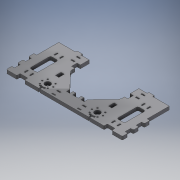
# Autodesk Inventor part: Bulkhead
Saved by Autodesk Inventor 2016 (Build 200138000, 138)
## iProperties
Created: 2014-06-30
Part Number: Bulkhead
Material: Generic
Document SubType Name: Modeling
Designer: STACKPOLE
Density: 1 g/cm^3
Appearance: Default
Author: STACKPOLE
Autodesk Inventor part; units mm, degrees
ref_plane "YZ Plane" through (0, 0, 0) normal (1, 0, 0) x (0, 1, 0)
ref_plane "XZ Plane" through (0, 0, 0) normal (0, 1, 0) x (-1, 0, 0)
ref_plane "XY Plane" through (0, 0, 0) normal (0, 0, 1) x (1, 0, 0)
sketch "Sketch1" plane through (0, 0, 0) normal (0, 0, 1) x (1, 0, 0)
  line L0 (0, -90) -> (-103, -90)
  line L1 (0, 0) -> (0, -90) construction
  line L2 (-105, -88) -> (-105, -82)
  line L3 (-103, -80) -> (-100, -80)
  line L4 (-100, -70) -> (-103, -70)
  line L5 (-105, -68) -> (-105, -62)
  line L6 (-103, -60) -> (-100, -60)
  line L7 (-100, -80) -> (-100, -70)
  line L8 (-100, -50) -> (-103, -50)
  line L9 (-105, -48) -> (-105, -42)
  line L10 (-103, -40) -> (-100, -40)
  line L11 (-100, -60) -> (-100, -50)
  line L12 (-100, -40) -> (-100, 0)
  line L13 (-70, 0) -> (-70, 3)
  line L14 (-70, 3) -> (-60, 3)
  line L15 (-60, 3) -> (-60, 0)
  line L16 (-100, 0) -> (-70, 0)
  line L17 (-60, 0) -> (-45, 0)
  line L18 (-45, 0) -> (-45, -29.9568)
  arc A0 (-105, -88) -> (-103, -90) centre (-103, -88) ccw
  arc A1 (-103, -80) -> (-105, -82) centre (-103, -82) ccw
  arc A2 (-105, -68) -> (-103, -70) centre (-103, -68) ccw
  arc A3 (-103, -60) -> (-105, -62) centre (-103, -62) ccw
  arc A4 (-105, -48) -> (-103, -50) centre (-103, -48) ccw
  arc A5 (-103, -40) -> (-105, -42) centre (-103, -42) ccw
  line L19 (0, -90) -> (103, -90)
  line L20 (105, -88) -> (105, -82)
  line L21 (103, -80) -> (100, -80)
  line L22 (100, -70) -> (103, -70)
  line L23 (105, -68) -> (105, -62)
  line L24 (103, -60) -> (100, -60)
  line L25 (100, -80) -> (100, -70)
  line L26 (100, -50) -> (103, -50)
  line L27 (105, -48) -> (105, -42)
  line L28 (103, -40) -> (100, -40)
  line L29 (100, -60) -> (100, -50)
  line L30 (100, -40) -> (100, 0)
  line L31 (70, 0) -> (70, 3)
  line L32 (70, 3) -> (60, 3)
  line L33 (60, 3) -> (60, 0)
  line L34 (100, 0) -> (70, 0)
  line L35 (60, 0) -> (45, 0)
  line L36 (45, 0) -> (45, -29.9568)
  arc A6 (103, -90) -> (105, -88) centre (103, -88) ccw
  arc A7 (105, -82) -> (103, -80) centre (103, -82) ccw
  arc A8 (103, -70) -> (105, -68) centre (103, -68) ccw
  arc A9 (105, -62) -> (103, -60) centre (103, -62) ccw
  arc A10 (103, -50) -> (105, -48) centre (103, -48) ccw
  arc A11 (105, -42) -> (103, -40) centre (103, -42) ccw
  line L37 (-42.1899, -36.907) -> (-16, -64)
  line L38 (16, -64) -> (42.1899, -36.907)
  line L39 (-16, -70) -> (-10, -70)
  line L40 (-10, -70) -> (-10, -64)
  line L41 (-5, -64) -> (-5, -70)
  line L42 (-5, -70) -> (5, -70)
  line L43 (5, -70) -> (5, -64)
  line L44 (10, -64) -> (10, -70)
  line L45 (10, -70) -> (16, -70)
  line L46 (-10, -64) -> (-5, -64)
  line L47 (5, -64) -> (10, -64)
  line L48 (16, -64) -> (16, -70)
  line L49 (-16, -64) -> (-16, -70)
  arc A12 (-45, -29.9568) -> (-42.1899, -36.907) centre (-35, -29.9568) ccw
  arc A13 (42.1899, -36.907) -> (45, -29.9568) centre (35, -29.9568) ccw
  point P0 (-105, -90)
  point P1 (-105, -80)
  point P2 (-105, -70)
  point P3 (-105, -60)
  point P4 (-105, -50)
  point P5 (-105, -40)
  point P6 (105, -90)
  point P7 (105, -80)
  point P8 (105, -70)
  point P9 (105, -60)
  point P10 (105, -50)
  point P11 (105, -40)
  point P12 (-45, -34)
  point P13 (45, -34)
  point P14 (0, -70)
  dimension "d4" = 105
  dimension "d5" = 10
  dimension "d6" = 5
  dimension "d8" = 10
  dimension "d9" = 10
  dimension "d10" = 10
  dimension "d11" = 10
  dimension "d12" = 30
  dimension "d13" = 10
  dimension "d14" = 3
  dimension "d15" = 90
  dimension "d18" = 15
  dimension "d19" = 34
  dimension "d20" = 2
  dimension "d102" = 5
  dimension "d104" = 5
  dimension "d105" = 10
  dimension "d160" = 6
  dimension "d161" = 6
  dimension "d162" = 6
  dimension "d163" = 70
  dimension "d175" = 10
  constraints: 100 end point, 36 symmetric about line, 28 point on circle, 28 point on line, 23 perpendicular, 16 tangent, 14 centre point, 10 parallel, 6 equal radius, 6 horizontal alignment, 5 vertical alignment, 2 horizontal, 1 midpoint, 1 vertical, 6 other
  measures "d4" distance of L0.start point (-105, -90)
  measures "d5" distance of point (-105, -90) point (-105, -80)
  measures "d6" distance of point (-105, -80) L3.end
  measures "d8" distance between parallel lines of L3 L4
  measures "d9" distance of point (-105, -70) point (-105, -60)
  measures "d10" distance between parallel lines of L6 L8
  measures "d11" distance of point (-105, -50) point (-105, -40)
  measures "d12" distance from line of L12 L13.start
  measures "d13" distance of L13.end L14.end
  measures "d14" distance of L13.start L13.end
  measures "d15" distance between parallel lines of L16 L0
  measures "d18" distance of L15.end L17.end
  measures "d19" distance of point (-45, -34) L17.end
  measures "d20" radius of A0
  measures "d102" distance between parallel lines of L41 L40
  measures "d104" distance between parallel lines of L44 L43
  measures "d105" distance between parallel lines of L41 L43
  measures "d160" distance of L37.end L39.start
  measures "d161" distance of L39.start L39.end
  measures "d162" distance of L44.end L45.end
  measures "d163" distance between parallel lines of L35 L42
  measures "d175" radius of A12
extrude "Extrusion1" add sketch "Sketch1" along normal blind 6
sketch "Sketch2" plane through (0, 0, 6) normal (0, 0, 1) x (1, 0, 0)
  line L0 (-103, -90) -> (103, -90) projected
  line L1 (-70, 0) -> (-100, 0) projected
  circle A0 centre (-45, -75) radius 5
  circle A1 centre (-45, -75) radius 10 construction
  line L2 (-45, -75) -> (-52.0711, -67.9289) construction
  line L3 (-45, -75) -> (-55, -75) construction
  line L4 (-55, -75) -> (-45, -75) construction
  circle A2 centre (-52.0711, -67.9289) radius 1.25
  circle A3 centre (-55, -75) radius 1.25
  circle A4 centre (-52.0711, -82.0711) radius 1.25
  line L5 (-45, -65) -> (-45, -85) construction
  circle A5 centre (-37.9289, -67.9289) radius 1.25
  circle A6 centre (-35, -75) radius 1.25
  circle A7 centre (-37.9289, -82.0711) radius 1.25
  line L6 (0, 0) -> (0, -90) construction
  circle A8 centre (45, -75) radius 5
  circle A9 centre (45, -75) radius 10 construction
  line L7 (45, -75) -> (52.0711, -67.9289) construction
  line L8 (45, -75) -> (55, -75) construction
  line L9 (55, -75) -> (45, -75) construction
  circle A10 centre (52.0711, -67.9289) radius 1.25
  circle A11 centre (55, -75) radius 1.25
  circle A12 centre (52.0711, -82.0711) radius 1.25
  line L10 (45, -65) -> (45, -85) construction
  circle A13 centre (37.9289, -67.9289) radius 1.25
  circle A14 centre (35, -75) radius 1.25
  circle A15 centre (37.9289, -82.0711) radius 1.25
  dimension "d23" = 10
  dimension "d25" = 75
  dimension "d26" = 45
  dimension "d27" = 20
  dimension "d28" = 45
  dimension "d29" = 2.5
  dimension "d30" = 2.5
  constraints: 18 end point, 16 centre point, 16 symmetric about line, 8 point on circle, 6 coincident, 1 collinear, 1 midpoint, 1 parallel, 1 perpendicular, 12 other
  measures "d23" diameter of A0
  measures "d25" vertical distance of A0.centre L6.start
  measures "d26" horizontal distance of L6.start A0.centre
  measures "d27" diameter of A1
  measures "d28" angle of L4 L2
  measures "d29" diameter of A2
  measures "d30" diameter of A3
extrude "Extrusion2" cut sketch "Sketch2" against normal blind 6
sketch "Sketch3" plane through (0, 0, 6) normal (0, 0, 1) x (1, 0, 0)
  line L0 (-103, -90) -> (103, -90) projected
  line L1 (-70, 0) -> (-100, 0) projected
  line L2 (-85, -18) -> (-83, -18)
  line L3 (-83, -18) -> (-83, -24)
  line L4 (-83, -24) -> (-85, -24)
  line L5 (-85, -24) -> (-85, -18)
  line L6 (-75, -18) -> (-73, -18)
  line L7 (-73, -18) -> (-73, -24)
  line L8 (-73, -24) -> (-75, -24)
  line L9 (-75, -24) -> (-75, -18)
  line L10 (0, 0) -> (0, -90) construction
  line L11 (85, -18) -> (83, -18)
  line L12 (83, -18) -> (83, -24)
  line L13 (83, -24) -> (85, -24)
  line L14 (85, -24) -> (85, -18)
  line L15 (75, -18) -> (73, -18)
  line L16 (73, -18) -> (73, -24)
  line L17 (73, -24) -> (75, -24)
  line L18 (75, -24) -> (75, -18)
  line L19 (-100, 0) -> (-100, -40) projected
  line L20 (-75, -21) -> (-83, -21) construction
  line L21 (-73, -78) -> (-75, -78)
  line L22 (-75, -78) -> (-75, -72)
  line L23 (-75, -72) -> (-73, -72)
  line L24 (-73, -72) -> (-73, -78)
  line L25 (-85, -72) -> (-83, -72)
  line L26 (-83, -72) -> (-83, -78)
  line L27 (-83, -78) -> (-85, -78)
  line L28 (-85, -78) -> (-85, -72)
  line L29 (73, -78) -> (75, -78)
  line L30 (75, -78) -> (75, -72)
  line L31 (75, -72) -> (73, -72)
  line L32 (73, -72) -> (73, -78)
  line L33 (85, -72) -> (83, -72)
  line L34 (83, -72) -> (83, -78)
  line L35 (83, -78) -> (85, -78)
  line L36 (85, -78) -> (85, -72)
  line L37 (-45, -29.9568) -> (-45, 0) projected
  line L38 (-55.5, -17) -> (-61.5, -17)
  line L39 (-61.5, -17) -> (-61.5, -15)
  line L40 (-61.5, -15) -> (-55.5, -15)
  line L41 (-55.5, -15) -> (-55.5, -17)
  line L42 (-55.5, -7) -> (-61.5, -7)
  line L43 (-61.5, -7) -> (-61.5, -5)
  line L44 (-61.5, -5) -> (-55.5, -5)
  line L45 (-55.5, -5) -> (-55.5, -7)
  line L46 (55.5, -17) -> (61.5, -17)
  line L47 (61.5, -17) -> (61.5, -15)
  line L48 (61.5, -15) -> (55.5, -15)
  line L49 (55.5, -15) -> (55.5, -17)
  line L50 (55.5, -7) -> (61.5, -7)
  line L51 (61.5, -7) -> (61.5, -5)
  line L52 (61.5, -5) -> (55.5, -5)
  line L53 (55.5, -5) -> (55.5, -7)
  point P0 (-79, -21)
  dimension "d41" = 6
  dimension "d43" = 18
  dimension "d129" = 15
  dimension "d130" = 8
  dimension "d131" = 2
  dimension "d132" = 2
  dimension "d219" = 12
  dimension "d314" = 5
  dimension "d316" = 8
  dimension "d317" = 10.5
  constraints: 100 end point, 24 symmetric about line, 12 parallel, 7 equal length, 6 horizontal, 6 perpendicular, 4 midpoint, 4 point on line, 3 collinear, 2 horizontal alignment
  measures "d41" distance of L4.end L2.start
  measures "d43" distance between parallel lines of L1 L2
  measures "d129" distance between parallel lines of L5 L19
  measures "d130" distance between parallel lines of L9 L3
  measures "d131" distance of L6.start L6.end
  measures "d132" distance of L2.start L2.end
  measures "d219" distance between parallel lines of L0 L27
  measures "d314" distance between parallel lines of L1 L44
  measures "d316" distance between parallel lines of L42 L40
  measures "d317" distance between parallel lines of L37 L41
sketch "Sketch8" plane through (0, 0, 6) normal (0, 0, 1) x (1, 0, 0)
  line L0 (-45, -29.9568) -> (-45, 0) projected
  line L1 (-45, -16) -> (-51, -16)
  line L2 (-51, -16) -> (-51, -26)
  line L3 (-51, -26) -> (-45, -26)
  line L4 (-45, -26) -> (-45, -16)
  line L5 (-45, 0) -> (-60, 0) projected
  line L6 (-45, -45) -> (-51, -45)
  line L7 (-51, -45) -> (-51, -55)
  line L8 (-51, -55) -> (-45, -55)
  line L9 (-45, -55) -> (-45, -45)
  line L10 (45, 0) -> (45, -29.9568) projected
  line L11 (45, -16) -> (51, -16)
  line L12 (51, -16) -> (51, -26)
  line L13 (51, -26) -> (45, -26)
  line L14 (45, -26) -> (45, -16)
  line L15 (45, -45) -> (51, -45)
  line L16 (51, -45) -> (51, -55)
  line L17 (51, -55) -> (45, -55)
  line L18 (45, -55) -> (45, -45)
  point P0 (0, 0)
  dimension "d177" = 6
  dimension "d178" = 10
  dimension "d179" = 16
  dimension "d180" = 10
  dimension "d181" = 6
  dimension "d182" = 55
  dimension "d183" = 6
  dimension "d184" = 10
  constraints: 32 end point, 8 parallel, 4 horizontal, 4 perpendicular, 3 horizontal alignment, 3 vertical alignment, 2 point on line
  measures "d177" distance of L1.start L1.end
  measures "d178" distance of L1.end L2.end
  measures "d179" distance between parallel lines of L5 L1
  measures "d180" distance of L6.end L7.end
  measures "d181" distance of L7.end L8.end
  measures "d182" distance between parallel lines of L5 L8
  measures "d183" distance of L11.start L11.end
  measures "d184" distance of L11.end L12.end
extrude "Extrusion16" cut sketch "Sketch8" against normal through all
sketch "Sketch9" plane through (0, 0, 6) normal (0, 0, 1) x (1, 0, 0)
  circle A0 centre (45, -75) radius 5 construction
  circle A1 centre (45, -75) radius 8.75 construction
  circle A2 centre (45, -75) radius 11.5 construction
  circle A3 centre (37.9289, -82.0711) radius 1.25 construction
  line L0 (-103, -90) -> (103, -90) construction
  line L1 (0, -90) -> (0, 0) construction
  line L2 (51, -45) -> (51, -55) projected
  arc A4 (40.8921, -82.7258) -> (49.1079, -82.7258) centre (45, -75) ccw
  line L3 (49.1079, -82.7258) -> (50.3989, -85.1539)
  line L4 (40.8921, -82.7258) -> (39.6011, -85.1539)
  line L5 (-103, -90) -> (103, -90) projected
  line L6 (45, -75) -> (45, -59.2152) construction
  line L7 (46.15, -90) -> (46.15, -86.4424)
  line L8 (43.85, -90) -> (43.85, -86.4424)
  arc A5 (39.6011, -85.1539) -> (43.85, -86.4424) centre (45, -75) ccw
  arc A6 (46.15, -86.4424) -> (50.3989, -85.1539) centre (45, -75) ccw
  line L9 (46.15, -90) -> (43.85, -90)
  circle A7 centre (-45, -75) radius 5 construction
  circle A8 centre (-45, -75) radius 8.75 construction
  circle A9 centre (-45, -75) radius 11.5 construction
  circle A10 centre (-37.9289, -82.0711) radius 1.25 construction
  line L10 (-51, -45) -> (-51, -55)
  arc A11 (-49.1079, -82.7258) -> (-40.8921, -82.7258) centre (-45, -75) ccw
  line L11 (-49.1079, -82.7258) -> (-50.3989, -85.1539)
  line L12 (-40.8921, -82.7258) -> (-39.6011, -85.1539)
  line L13 (-45, -75) -> (-45, -59.2152) construction
  line L14 (-46.15, -90) -> (-46.15, -86.4424)
  line L15 (-43.85, -90) -> (-43.85, -86.4424)
  arc A12 (-43.85, -86.4424) -> (-39.6011, -85.1539) centre (-45, -75) ccw
  arc A13 (-50.3989, -85.1539) -> (-46.15, -86.4424) centre (-45, -75) ccw
  line L16 (-46.15, -90) -> (-43.85, -90)
  point P0 (77, -74)
  point P1 (79, -74)
  point P2 (46.7957, -86.3589)
  point P3 (44, -86.4564)
  point P4 (-46.7957, -86.3589)
  point P5 (-44, -86.4564)
  dimension "d191" = 23
  dimension "d239" = 56
  dimension "d288" = 28
  dimension "d289" = 2.3
  dimension "d290" = 1.15
  constraints: 28 end point, 28 point on circle, 19 symmetric about line, 12 centre point, 4 coincident, 4 line through centre, 2 point on line, 2 vertical, 1 collinear, 1 concentric, 1 midpoint, 1 parallel, 1 perpendicular, 1 tangent, 7 other
  measures "d191" diameter of A2
  measures "d239" angle of L4 L3
  measures "d288" angle of L6 L4
  measures "d289" distance between parallel lines of L8 L7
  measures "d290" distance between parallel lines of L8 L6
extrude "Extrusion31" cut sketch "Sketch3" against normal through all
extrude "Extrusion32" cut sketch "Sketch9" against normal blind 10
sketch "Sketch20" plane through (0, 0, 6) normal (0, 0, 1) x (1, 0, 0)
  line L0 (0, 0) -> (0, -123) construction
  line L1 (-20, -87) -> (-26, -87)
  line L2 (-26, -87) -> (-26, -85)
  line L3 (-26, -85) -> (-20, -85)
  line L4 (-20, -85) -> (-20, -87)
  line L5 (-20, -78) -> (-26, -78)
  line L6 (-26, -78) -> (-26, -76)
  line L7 (-26, -76) -> (-20, -76)
  line L8 (-20, -76) -> (-20, -78)
  line L9 (-43.85, -90) -> (43.85, -90) projected
  line L10 (20, -87) -> (26, -87)
  line L11 (26, -87) -> (26, -85)
  line L12 (26, -85) -> (20, -85)
  line L13 (20, -85) -> (20, -87)
  line L14 (20, -78) -> (26, -78)
  line L15 (26, -78) -> (26, -76)
  line L16 (26, -76) -> (20, -76)
  line L17 (20, -76) -> (20, -78)
  dimension "d293" = 2
  dimension "d294" = 2
  dimension "d295" = 7
  dimension "d296" = 6
  dimension "d297" = 3
  dimension "d298" = 20
  constraints: 34 end point, 8 symmetric about line, 4 parallel, 2 horizontal, 2 perpendicular, 2 point on line, 1 collinear, 1 vertical
  measures "d293" distance of L1.end L2.end
  measures "d294" distance of L5.end L6.end
  measures "d295" distance between parallel lines of L5 L3
  measures "d296" distance of L1.start L1.end
  measures "d297" distance between parallel lines of L9 L1
  measures "d298" distance between parallel lines of L0 L4
extrude "Extrusion33" cut sketch "Sketch20" against normal blind 10
sketch "Sketch21" plane through (0, 0, 6) normal (0, 0, 1) x (1, 0, 0)
  line L0 (83, -67) -> (75, -67)
  line L1 (72, -64) -> (72, -32)
  line L2 (75, -29) -> (83, -29)
  line L3 (86, -32) -> (86, -64)
  line L4 (85, -72) -> (85, -78) projected
  line L5 (73, -78) -> (73, -72) projected
  line L6 (75, -72) -> (73, -72) projected
  line L7 (75, -24) -> (73, -24) projected
  arc A0 (83, -67) -> (86, -64) centre (83, -64) ccw
  arc A1 (72, -64) -> (75, -67) centre (75, -64) ccw
  arc A2 (75, -29) -> (72, -32) centre (75, -32) ccw
  arc A3 (86, -32) -> (83, -29) centre (83, -32) ccw
  line L8 (0, 0) -> (0, -90) construction
  line L9 (-43.85, -90) -> (43.85, -90) construction
  line L10 (-83, -67) -> (-75, -67)
  line L11 (-72, -64) -> (-72, -32)
  line L12 (-75, -29) -> (-83, -29)
  line L13 (-86, -32) -> (-86, -64)
  arc A4 (-86, -64) -> (-83, -67) centre (-83, -64) ccw
  arc A5 (-75, -67) -> (-72, -64) centre (-75, -64) ccw
  arc A6 (-72, -32) -> (-75, -29) centre (-75, -32) ccw
  arc A7 (-83, -29) -> (-86, -32) centre (-83, -32) ccw
  line L14 (83, -72) -> (83, -78) construction
  line L15 (83, -75) -> (75, -75) construction
  line L16 (75, -72) -> (75, -78) construction
  point P0 (79, -67)
  point P1 (79, -75)
  dimension "d301" = 5
  dimension "d302" = 5
  dimension "d303" = 3
  dimension "d310" = 14
  constraints: 20 end point, 16 point on circle, 12 symmetric about line, 8 centre point, 8 tangent, 5 midpoint, 3 equal radius, 2 parallel, 1 horizontal, 1 perpendicular, 1 vertical alignment, 4 other
  measures "d301" distance between parallel lines of L6 L0
  measures "d302" distance between parallel lines of L7 L2
  measures "d303" radius of A0
  measures "d310" distance between parallel lines of L1 L3
extrude "Extrusion34" cut sketch "Sketch21" against normal through all
sketch "Sketch22" plane through (0, 0, 6) normal (0, 0, 1) x (1, 0, 0)
  line L0 (46.15, -90) -> (103, -90) projected
  line L1 (86, -90) -> (86, -84)
  line L2 (86, -84) -> (72, -84)
  line L3 (72, -84) -> (72, -90)
  line L4 (-103, -90) -> (-46.15, -90) projected
  line L5 (-72, -84) -> (-86, -84)
  line L6 (-86, -84) -> (-86, -90)
  line L7 (-86, -64) -> (-86, -32) projected
  line L8 (-72, -84) -> (-72, -90)
  line L9 (-72, -32) -> (-72, -64) projected
  line L10 (72, -64) -> (72, -32) projected
  line L11 (86, -32) -> (86, -64) projected
  point P0 (0, 0)
  dimension "d306" = 6
  constraints: 12 end point, 5 collinear, 4 perpendicular, 4 point on line, 1 parallel, 1 vertical
  measures "d306" distance between parallel lines of L0 L2
extrude "Extrusion35" cut sketch "Sketch22" against normal through all
fillet "Fillet10" radius 1.5 6 edges at (86, -90, 3) (86, -84, 3) (72, -84, 3) (72, -90, 3) (-72, -84, 3) (-86, -84, 3)
body "Solid1"
